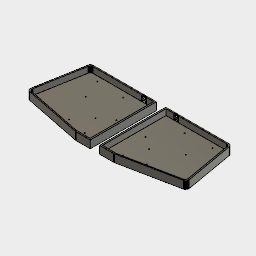
Split 62 bot (Autodesk Fusion 360 design; units mm, degrees)
Autodesk Fusion 360 part; units mm, degrees
note: some values were not read from the file. Chosen so that the rebuilt part matches the saved one: which pieces of a blend or face edit are solid. Set by a fixed rule: which sketch regions a step uses.
(part 1 of 2)
sketch "Sketch1" plane through (0, 0, 0) normal (0, 1, 0) x (1, 0, 0)
  line L0 (21.6572, -133.3169) -> (140.5792, -109.2975)
  line L1 (-8.8048, -133.4855) -> (-8.8048, 3.2554)
  line L2 (-8.8048, 3.2554) -> (-8.8048, -133.4855)
  line L3 (-8.8048, -133.4855) -> (20.1607, -133.4847)
  line L4 (20.1607, -133.4847) -> (20.9148, -133.4484)
  line L5 (20.9148, -133.4484) -> (20.9148, -133.4492)
  line L6 (20.9148, -133.4492) -> (21.658, -133.3177)
  line L7 (21.658, -133.3177) -> (140.5792, -109.2975)
  line L8 (140.5792, -109.2975) -> (141.2999, -109.074)
  line L9 (141.2999, -109.074) -> (141.9873, -108.7628)
  line L10 (141.9873, -108.7628) -> (141.9873, -108.7636)
  line L11 (141.9873, -108.7636) -> (142.6297, -108.368)
  line L12 (142.6297, -108.368) -> (142.6297, -108.3675)
  line L13 (142.6297, -108.3675) -> (143.2182, -107.8942)
  line L14 (143.2182, -107.8942) -> (143.2182, -107.8947)
  line L15 (143.2182, -107.8947) -> (143.7407, -107.3526)
  line L16 (143.7407, -107.3526) -> (143.742, -107.3518)
  line L17 (143.742, -107.3518) -> (144.1939, -106.7475)
  line L18 (144.1939, -106.7475) -> (144.567, -106.0918)
  line L19 (144.567, -106.0918) -> (144.8541, -105.3933)
  line L20 (144.8541, -105.3933) -> (145.0515, -104.6655)
  line L21 (145.0515, -104.6655) -> (145.0515, -104.6668)
  line L22 (145.0515, -104.6668) -> (145.157, -103.9196)
  line L23 (145.157, -103.9196) -> (145.1568, -103.9191)
  line L24 (145.1568, -103.9191) -> (145.1676, -103.1642)
  line L25 (145.1676, -103.1642) -> (145.1681, -103.165)
  line L26 (145.1681, -103.165) -> (145.0837, -102.4157)
  line L27 (145.0837, -102.4157) -> (127.3268, -1.7092)
  line L28 (127.3268, -1.7092) -> (127.1498, -0.9763)
  line L29 (127.1498, -0.9763) -> (126.8809, -0.2707)
  line L30 (126.8809, -0.2707) -> (126.5264, 0.3956)
  line L31 (126.5264, 0.3956) -> (126.0917, 1.0126)
  line L32 (126.0917, 1.0126) -> (125.584, 1.569)
  line L33 (125.584, 1.569) -> (125.5832, 1.569)
  line L34 (125.5832, 1.569) -> (125.008, 2.0577)
  line L35 (125.008, 2.0577) -> (124.3769, 2.4712)
  line L36 (124.3769, 2.4712) -> (123.698, 2.8022)
  line L37 (123.698, 2.8022) -> (122.9839, 3.0454)
  line L38 (122.9839, 3.0454) -> (122.9847, 3.0454)
  line L39 (122.9847, 3.0454) -> (122.2457, 3.1975)
  line L40 (122.2457, 3.1975) -> (121.4935, 3.2554)
  line L41 (-8.8048, 3.2554) -> (121.4935, 3.2554)
  line L42 (121.4935, 3.2554) -> (-8.8048, 3.2554)
  line L43 (20.9619, -101.3068) -> (36.3252, -98.5991)
  line L44 (36.3252, -98.5991) -> (34.1021, -85.9914)
  line L45 (34.1021, -85.9914) -> (18.7391, -88.7016)
  line L46 (18.7391, -88.7016) -> (20.9619, -101.3068)
  line L47 (17.6538, -82.5463) -> (33.0171, -79.8372)
  line L48 (33.0171, -79.8372) -> (30.7935, -67.233)
  line L49 (30.7935, -67.233) -> (15.4313, -69.9413)
  line L50 (15.4313, -69.9413) -> (17.6538, -82.5463)
  line L51 (14.3452, -63.7865) -> (29.709, -61.0775)
  line L52 (29.709, -61.0775) -> (27.4862, -48.4717)
  line L53 (27.4862, -48.4717) -> (12.1232, -51.1802)
  line L54 (12.1232, -51.1802) -> (14.3452, -63.7865)
  line L55 (11.0379, -45.0257) -> (26.4012, -42.3164)
  line L56 (26.4012, -42.3164) -> (24.1774, -29.7116)
  line L57 (24.1774, -29.7116) -> (8.8151, -32.4207)
  line L58 (8.8151, -32.4207) -> (11.0379, -45.0257)
  line L59 (24.3242, -119.9698) -> (39.6867, -117.2604)
  line L60 (39.6867, -117.2604) -> (37.4645, -104.6549)
  line L61 (37.4645, -104.6549) -> (22.1017, -107.3634)
  line L62 (22.1017, -107.3634) -> (24.3242, -119.9698)
  line L63 (38.8681, -92.991) -> (54.2311, -90.2819)
  line L64 (54.2311, -90.2819) -> (52.0084, -77.6764)
  line L65 (52.0084, -77.6764) -> (36.6453, -80.3857)
  line L66 (36.6453, -80.3857) -> (38.8681, -92.991)
  line L67 (35.4976, -74.2789) -> (50.8611, -71.5698)
  line L68 (50.8611, -71.5698) -> (48.6386, -58.965)
  line L69 (48.6386, -58.965) -> (33.2753, -61.6744)
  line L70 (33.2753, -61.6744) -> (35.4976, -74.2789)
  line L71 (32.2686, -55.5432) -> (47.6319, -52.8341)
  line L72 (47.6319, -52.8341) -> (45.4091, -40.2278)
  line L73 (45.4091, -40.2278) -> (30.0458, -42.9371)
  line L74 (30.0458, -42.9371) -> (32.2686, -55.5432)
  line L75 (28.8147, -36.8768) -> (44.1777, -34.1678)
  line L76 (44.1777, -34.1678) -> (41.9542, -21.563)
  line L77 (41.9542, -21.563) -> (26.5917, -24.2718)
  line L78 (26.5917, -24.2718) -> (28.8147, -36.8768)
  line L79 (42.1672, -111.7235) -> (57.5302, -109.0136)
  line L80 (57.5302, -109.0136) -> (55.3074, -96.4076)
  line L81 (55.3074, -96.4076) -> (39.9444, -99.1166)
  line L82 (39.9444, -99.1166) -> (42.1672, -111.7235)
  line L83 (56.5505, -83.8047) -> (71.9135, -81.0951)
  line L84 (71.9135, -81.0951) -> (69.6907, -68.489)
  line L85 (69.6907, -68.489) -> (54.3272, -71.1981)
  line L86 (54.3272, -71.1981) -> (56.5505, -83.8047)
  line L87 (53.2424, -65.1431) -> (68.6054, -62.4337)
  line L88 (68.6054, -62.4337) -> (66.3826, -49.8292)
  line L89 (66.3826, -49.8292) -> (51.0199, -52.5386)
  line L90 (51.0199, -52.5386) -> (53.2424, -65.1431)
  line L91 (49.9345, -46.383) -> (65.2973, -43.6742)
  line L92 (65.2973, -43.6742) -> (63.0748, -31.0679)
  line L93 (63.0748, -31.0679) -> (47.7118, -33.7772)
  line L94 (47.7118, -33.7772) -> (49.9345, -46.383)
  line L95 (46.6265, -27.6222) -> (61.9898, -24.9132)
  line L96 (61.9898, -24.9132) -> (59.7659, -12.3084)
  line L97 (59.7659, -12.3084) -> (44.4037, -15.0175)
  line L98 (44.4037, -15.0175) -> (46.6265, -27.6222)
  line L99 (59.7847, -102.5155) -> (75.1478, -99.8061)
  line L100 (75.1478, -99.8061) -> (72.925, -87.2001)
  line L101 (72.925, -87.2001) -> (57.5612, -89.9091)
  line L102 (57.5612, -89.9091) -> (59.7847, -102.5155)
  line L103 (76.1309, -85.4056) -> (91.494, -82.6966)
  line L104 (91.494, -82.6966) -> (89.2712, -70.091)
  line L105 (89.2712, -70.091) -> (73.9082, -72.8001)
  line L106 (73.9082, -72.8001) -> (76.1309, -85.4056)
  line L107 (72.8231, -66.6454) -> (88.1859, -63.9366)
  line L108 (88.1859, -63.9366) -> (85.9634, -51.3313)
  line L109 (85.9634, -51.3313) -> (70.5996, -54.0406)
  line L110 (70.5996, -54.0406) -> (72.8231, -66.6454)
  line L111 (69.515, -47.8859) -> (84.8781, -45.1765)
  line L112 (84.8781, -45.1765) -> (82.6553, -32.5705)
  line L113 (82.6553, -32.5705) -> (67.2917, -35.2795)
  line L114 (67.2917, -35.2795) -> (69.515, -47.8859)
  line L115 (66.207, -29.2428) -> (81.57, -26.534)
  line L116 (81.57, -26.534) -> (79.3467, -13.9287)
  line L117 (79.3467, -13.9287) -> (63.9837, -16.6373)
  line L118 (63.9837, -16.6373) -> (66.207, -29.2428)
  line L119 (79.3644, -104.2064) -> (94.7277, -101.4965)
  line L120 (94.7277, -101.4965) -> (92.5049, -88.8899)
  line L121 (92.5049, -88.8899) -> (77.1417, -91.6001)
  line L122 (77.1417, -91.6001) -> (79.3644, -104.2064)
  line L123 (95.3622, -85.0606) -> (110.7252, -82.3516)
  line L124 (110.7252, -82.3516) -> (108.5025, -69.745)
  line L125 (108.5025, -69.745) -> (93.1394, -72.4543)
  line L126 (93.1394, -72.4543) -> (95.3622, -85.0606)
  line L127 (92.0541, -66.2993) -> (107.4174, -63.5908)
  line L128 (107.4174, -63.5908) -> (105.1944, -50.9857)
  line L129 (105.1944, -50.9857) -> (89.8313, -53.6948)
  line L130 (89.8313, -53.6948) -> (92.0541, -66.2993)
  line L131 (88.746, -47.5401) -> (104.1093, -44.8302)
  line L132 (104.1093, -44.8302) -> (101.8865, -32.2247)
  line L133 (101.8865, -32.2247) -> (86.5235, -34.9337)
  line L134 (86.5235, -34.9337) -> (88.746, -47.5401)
  line L135 (85.4385, -28.8973) -> (100.8012, -26.1885)
  line L136 (100.8012, -26.1885) -> (98.5787, -13.5834)
  line L137 (98.5787, -13.5834) -> (83.2154, -16.2925)
  line L138 (83.2154, -16.2925) -> (85.4385, -28.8973)
  line L139 (98.5965, -103.8611) -> (113.9587, -101.1513)
  line L140 (113.9587, -101.1513) -> (111.7367, -88.5449)
  line L141 (111.7367, -88.5449) -> (96.3737, -91.2543)
  line L142 (96.3737, -91.2543) -> (98.5965, -103.8611)
  line L143 (114.0738, -81.6816) -> (129.4368, -78.9723)
  line L144 (129.4368, -78.9723) -> (127.214, -66.3662)
  line L145 (127.214, -66.3662) -> (111.8513, -69.0753)
  line L146 (111.8513, -69.0753) -> (114.0738, -81.6816)
  line L147 (110.766, -62.9211) -> (126.129, -60.2123)
  line L148 (126.129, -60.2123) -> (123.9062, -47.607)
  line L149 (123.9062, -47.607) -> (108.5432, -50.3163)
  line L150 (108.5432, -50.3163) -> (110.766, -62.9211)
  line L151 (107.4579, -44.3008) -> (122.8212, -41.5917)
  line L152 (122.8212, -41.5917) -> (120.5981, -28.9859)
  line L153 (120.5981, -28.9859) -> (105.2351, -31.695)
  line L154 (105.2351, -31.695) -> (107.4579, -44.3008)
  line L155 (104.2464, -25.5889) -> (119.6094, -22.8804)
  line L156 (119.6094, -22.8804) -> (117.3861, -10.2754)
  line L157 (117.3861, -10.2754) -> (102.0236, -12.9842)
  line L158 (102.0236, -12.9842) -> (104.2464, -25.5889)
  line L159 (117.3075, -100.4816) -> (132.6706, -97.7731)
  line L160 (132.6706, -97.7731) -> (130.4478, -85.1659)
  line L161 (130.4478, -85.1659) -> (115.0845, -87.875)
  line L162 (115.0845, -87.875) -> (117.3075, -100.4816)
  line L163 (3.9632, -113.914) -> (19.326, -111.2038)
  line L164 (19.326, -111.2038) -> (17.1035, -98.5986)
  line L165 (17.1035, -98.5986) -> (1.7404, -101.3063)
  line L166 (1.7404, -101.3063) -> (3.9632, -113.914)
  line L167 (19.6816, -136.2128) -> (143.6531, -111.1734)
  line L168 (-12.0737, -136.3885) -> (-12.0737, 6.1587)
  line L169 (-12.0737, 6.1587) -> (-12.0737, -136.3885)
  line L170 (-12.0737, -136.3885) -> (18.1216, -136.3877)
  line L171 (18.1216, -136.3877) -> (18.9079, -136.3493)
  line L172 (18.9079, -136.3493) -> (18.9079, -136.3501)
  line L173 (18.9079, -136.3501) -> (19.6824, -136.2139)
  line L174 (19.6824, -136.2139) -> (143.6531, -111.1734)
  line L175 (143.6531, -111.1734) -> (144.4046, -110.9403)
  line L176 (144.4046, -110.9403) -> (145.121, -110.6159)
  line L177 (145.121, -110.6159) -> (145.121, -110.6167)
  line L178 (145.121, -110.6167) -> (145.7907, -110.2045)
  line L179 (145.7907, -110.2045) -> (145.7907, -110.204)
  line L180 (145.7907, -110.204) -> (146.4043, -109.7103)
  line L181 (146.4043, -109.7103) -> (146.4043, -109.7113)
  line L182 (146.4043, -109.7113) -> (146.9488, -109.1457)
  line L183 (146.9488, -109.1457) -> (146.9501, -109.1449)
  line L184 (146.9501, -109.1449) -> (147.4213, -108.5146)
  line L185 (147.4213, -108.5146) -> (147.8108, -107.8315)
  line L186 (147.8108, -107.8315) -> (148.1098, -107.1036)
  line L187 (148.1098, -107.1036) -> (148.3154, -106.3448)
  line L188 (148.3154, -106.3448) -> (148.3154, -106.3461)
  line L189 (148.3154, -106.3461) -> (148.4257, -105.5672)
  line L190 (148.4257, -105.5672) -> (148.4249, -105.5666)
  line L191 (148.4249, -105.5666) -> (148.4363, -104.7795)
  line L192 (148.4363, -104.7795) -> (148.4371, -104.7803)
  line L193 (148.4371, -104.7803) -> (148.3492, -103.9992)
  line L194 (148.3492, -103.9992) -> (129.8382, 0.9829)
  line L195 (129.8382, 0.9829) -> (129.6532, 1.7473)
  line L196 (129.6532, 1.7473) -> (129.3736, 2.4831)
  line L197 (129.3736, 2.4831) -> (129.004, 3.1771)
  line L198 (129.004, 3.1771) -> (128.5505, 3.8201)
  line L199 (128.5505, 3.8201) -> (128.0213, 4.4006)
  line L200 (128.0213, 4.4006) -> (128.0208, 4.4006)
  line L201 (128.0208, 4.4006) -> (127.4204, 4.9101)
  line L202 (127.4204, 4.9101) -> (126.7632, 5.3411)
  line L203 (126.7632, 5.3411) -> (126.0554, 5.6864)
  line L204 (126.0554, 5.6864) -> (125.3112, 5.9396)
  line L205 (125.3112, 5.9396) -> (125.312, 5.9396)
  line L206 (125.312, 5.9396) -> (124.5415, 6.0984)
  line L207 (124.5415, 6.0984) -> (123.7575, 6.1587)
  line L208 (-12.0737, 6.1587) -> (123.7575, 6.1587)
  line L209 (123.7575, 6.1587) -> (-12.0737, 6.1587)
extrude "Extrude1" add sketch "Sketch1" along normal blind 16.7 contours L167 L168 L169 L170 L171 L173 L174 L175 L176 L178 L180 L182 L184 L185 L186 L187 L189 L191 L193 L194 L195 L196 L197 L198 L199 L201 L202 L203 L204 L206 L207 L208 L209 makes body 1
sketch "Sketch2" plane through (0, 0, 0) normal (0, 1, 0) x (1, 0, 0)
  line L0 (21.6572, -133.3169) -> (140.5792, -109.2975)
  line L1 (-8.8048, -133.4855) -> (-8.8048, 3.2554)
  line L2 (-8.8048, 3.2554) -> (-8.8048, -133.4855)
  line L3 (-8.8048, -133.4855) -> (20.1607, -133.4847)
  line L4 (20.1607, -133.4847) -> (20.9148, -133.4484)
  line L5 (20.9148, -133.4484) -> (20.9148, -133.4492)
  line L6 (20.9148, -133.4492) -> (21.658, -133.3177)
  line L7 (21.658, -133.3177) -> (140.5792, -109.2975)
  line L8 (140.5792, -109.2975) -> (141.2999, -109.074)
  line L9 (141.2999, -109.074) -> (141.9873, -108.7628)
  line L10 (141.9873, -108.7628) -> (141.9873, -108.7636)
  line L11 (141.9873, -108.7636) -> (142.6297, -108.368)
  line L12 (142.6297, -108.368) -> (142.6297, -108.3675)
  line L13 (142.6297, -108.3675) -> (143.2182, -107.8942)
  line L14 (143.2182, -107.8942) -> (143.2182, -107.8947)
  line L15 (143.2182, -107.8947) -> (143.7407, -107.3526)
  line L16 (143.7407, -107.3526) -> (143.742, -107.3518)
  line L17 (143.742, -107.3518) -> (144.1939, -106.7475)
  line L18 (144.1939, -106.7475) -> (144.567, -106.0918)
  line L19 (144.567, -106.0918) -> (144.8541, -105.3933)
  line L20 (144.8541, -105.3933) -> (145.0515, -104.6655)
  line L21 (145.0515, -104.6655) -> (145.0515, -104.6668)
  line L22 (145.0515, -104.6668) -> (145.157, -103.9196)
  line L23 (145.157, -103.9196) -> (145.1568, -103.9191)
  line L24 (145.1568, -103.9191) -> (145.1676, -103.1642)
  line L25 (145.1676, -103.1642) -> (145.1681, -103.165)
  line L26 (145.1681, -103.165) -> (145.0837, -102.4157)
  line L27 (145.0837, -102.4157) -> (127.3268, -1.7092)
  line L28 (127.3268, -1.7092) -> (127.1498, -0.9763)
  line L29 (127.1498, -0.9763) -> (126.8809, -0.2707)
  line L30 (126.8809, -0.2707) -> (126.5264, 0.3956)
  line L31 (126.5264, 0.3956) -> (126.0917, 1.0126)
  line L32 (126.0917, 1.0126) -> (125.584, 1.569)
  line L33 (125.584, 1.569) -> (125.5832, 1.569)
  line L34 (125.5832, 1.569) -> (125.008, 2.0577)
  line L35 (125.008, 2.0577) -> (124.3769, 2.4712)
  line L36 (124.3769, 2.4712) -> (123.698, 2.8022)
  line L37 (123.698, 2.8022) -> (122.9839, 3.0454)
  line L38 (122.9839, 3.0454) -> (122.9847, 3.0454)
  line L39 (122.9847, 3.0454) -> (122.2457, 3.1975)
  line L40 (122.2457, 3.1975) -> (121.4935, 3.2554)
  line L41 (-8.8048, 3.2554) -> (121.4935, 3.2554)
  line L42 (121.4935, 3.2554) -> (-8.8048, 3.2554)
  line L43 (20.9619, -101.3068) -> (36.3252, -98.5991)
  line L44 (36.3252, -98.5991) -> (34.1021, -85.9914)
  line L45 (34.1021, -85.9914) -> (18.7391, -88.7016)
  line L46 (18.7391, -88.7016) -> (20.9619, -101.3068)
  line L47 (17.6538, -82.5463) -> (33.0171, -79.8372)
  line L48 (33.0171, -79.8372) -> (30.7935, -67.233)
  line L49 (30.7935, -67.233) -> (15.4313, -69.9413)
  line L50 (15.4313, -69.9413) -> (17.6538, -82.5463)
  line L51 (14.3452, -63.7865) -> (29.709, -61.0775)
  line L52 (29.709, -61.0775) -> (27.4862, -48.4717)
  line L53 (27.4862, -48.4717) -> (12.1232, -51.1802)
  line L54 (12.1232, -51.1802) -> (14.3452, -63.7865)
  line L55 (11.0379, -45.0257) -> (26.4012, -42.3164)
  line L56 (26.4012, -42.3164) -> (24.1774, -29.7116)
  line L57 (24.1774, -29.7116) -> (8.8151, -32.4207)
  line L58 (8.8151, -32.4207) -> (11.0379, -45.0257)
  line L59 (24.3242, -119.9698) -> (39.6867, -117.2604)
  line L60 (39.6867, -117.2604) -> (37.4645, -104.6549)
  line L61 (37.4645, -104.6549) -> (22.1017, -107.3634)
  line L62 (22.1017, -107.3634) -> (24.3242, -119.9698)
  line L63 (38.8681, -92.991) -> (54.2311, -90.2819)
  line L64 (54.2311, -90.2819) -> (52.0084, -77.6764)
  line L65 (52.0084, -77.6764) -> (36.6453, -80.3857)
  line L66 (36.6453, -80.3857) -> (38.8681, -92.991)
  line L67 (35.4976, -74.2789) -> (50.8611, -71.5698)
  line L68 (50.8611, -71.5698) -> (48.6386, -58.965)
  line L69 (48.6386, -58.965) -> (33.2753, -61.6744)
  line L70 (33.2753, -61.6744) -> (35.4976, -74.2789)
  line L71 (32.2686, -55.5432) -> (47.6319, -52.8341)
  line L72 (47.6319, -52.8341) -> (45.4091, -40.2278)
  line L73 (45.4091, -40.2278) -> (30.0458, -42.9371)
  line L74 (30.0458, -42.9371) -> (32.2686, -55.5432)
  line L75 (28.8147, -36.8768) -> (44.1777, -34.1678)
  line L76 (44.1777, -34.1678) -> (41.9542, -21.563)
  line L77 (41.9542, -21.563) -> (26.5917, -24.2718)
  line L78 (26.5917, -24.2718) -> (28.8147, -36.8768)
  line L79 (42.1672, -111.7235) -> (57.5302, -109.0136)
  line L80 (57.5302, -109.0136) -> (55.3074, -96.4076)
  line L81 (55.3074, -96.4076) -> (39.9444, -99.1166)
  line L82 (39.9444, -99.1166) -> (42.1672, -111.7235)
  line L83 (56.5505, -83.8047) -> (71.9135, -81.0951)
  line L84 (71.9135, -81.0951) -> (69.6907, -68.489)
  line L85 (69.6907, -68.489) -> (54.3272, -71.1981)
  line L86 (54.3272, -71.1981) -> (56.5505, -83.8047)
  line L87 (53.2424, -65.1431) -> (68.6054, -62.4337)
  line L88 (68.6054, -62.4337) -> (66.3826, -49.8292)
  line L89 (66.3826, -49.8292) -> (51.0199, -52.5386)
  line L90 (51.0199, -52.5386) -> (53.2424, -65.1431)
  line L91 (49.9345, -46.383) -> (65.2973, -43.6742)
  line L92 (65.2973, -43.6742) -> (63.0748, -31.0679)
  line L93 (63.0748, -31.0679) -> (47.7118, -33.7772)
  line L94 (47.7118, -33.7772) -> (49.9345, -46.383)
  line L95 (46.6265, -27.6222) -> (61.9898, -24.9132)
  line L96 (61.9898, -24.9132) -> (59.7659, -12.3084)
  line L97 (59.7659, -12.3084) -> (44.4037, -15.0175)
  line L98 (44.4037, -15.0175) -> (46.6265, -27.6222)
  line L99 (59.7847, -102.5155) -> (75.1478, -99.8061)
  line L100 (75.1478, -99.8061) -> (72.925, -87.2001)
  line L101 (72.925, -87.2001) -> (57.5612, -89.9091)
  line L102 (57.5612, -89.9091) -> (59.7847, -102.5155)
  line L103 (76.1309, -85.4056) -> (91.494, -82.6966)
  line L104 (91.494, -82.6966) -> (89.2712, -70.091)
  line L105 (89.2712, -70.091) -> (73.9082, -72.8001)
  line L106 (73.9082, -72.8001) -> (76.1309, -85.4056)
  line L107 (72.8231, -66.6454) -> (88.1859, -63.9366)
  line L108 (88.1859, -63.9366) -> (85.9634, -51.3313)
  line L109 (85.9634, -51.3313) -> (70.5996, -54.0406)
  line L110 (70.5996, -54.0406) -> (72.8231, -66.6454)
  line L111 (69.515, -47.8859) -> (84.8781, -45.1765)
  line L112 (84.8781, -45.1765) -> (82.6553, -32.5705)
  line L113 (82.6553, -32.5705) -> (67.2917, -35.2795)
  line L114 (67.2917, -35.2795) -> (69.515, -47.8859)
  line L115 (66.207, -29.2428) -> (81.57, -26.534)
  line L116 (81.57, -26.534) -> (79.3467, -13.9287)
  line L117 (79.3467, -13.9287) -> (63.9837, -16.6373)
  line L118 (63.9837, -16.6373) -> (66.207, -29.2428)
  line L119 (79.3644, -104.2064) -> (94.7277, -101.4965)
  line L120 (94.7277, -101.4965) -> (92.5049, -88.8899)
  line L121 (92.5049, -88.8899) -> (77.1417, -91.6001)
  line L122 (77.1417, -91.6001) -> (79.3644, -104.2064)
  line L123 (95.3622, -85.0606) -> (110.7252, -82.3516)
  line L124 (110.7252, -82.3516) -> (108.5025, -69.745)
  line L125 (108.5025, -69.745) -> (93.1394, -72.4543)
  line L126 (93.1394, -72.4543) -> (95.3622, -85.0606)
  line L127 (92.0541, -66.2993) -> (107.4174, -63.5908)
  line L128 (107.4174, -63.5908) -> (105.1944, -50.9857)
  line L129 (105.1944, -50.9857) -> (89.8313, -53.6948)
  line L130 (89.8313, -53.6948) -> (92.0541, -66.2993)
  line L131 (88.746, -47.5401) -> (104.1093, -44.8302)
  line L132 (104.1093, -44.8302) -> (101.8865, -32.2247)
  line L133 (101.8865, -32.2247) -> (86.5235, -34.9337)
  line L134 (86.5235, -34.9337) -> (88.746, -47.5401)
  line L135 (85.4385, -28.8973) -> (100.8012, -26.1885)
  line L136 (100.8012, -26.1885) -> (98.5787, -13.5834)
  line L137 (98.5787, -13.5834) -> (83.2154, -16.2925)
  line L138 (83.2154, -16.2925) -> (85.4385, -28.8973)
  line L139 (98.5965, -103.8611) -> (113.9587, -101.1513)
  line L140 (113.9587, -101.1513) -> (111.7367, -88.5449)
  line L141 (111.7367, -88.5449) -> (96.3737, -91.2543)
  line L142 (96.3737, -91.2543) -> (98.5965, -103.8611)
  line L143 (114.0738, -81.6816) -> (129.4368, -78.9723)
  line L144 (129.4368, -78.9723) -> (127.214, -66.3662)
  line L145 (127.214, -66.3662) -> (111.8513, -69.0753)
  line L146 (111.8513, -69.0753) -> (114.0738, -81.6816)
  line L147 (110.766, -62.9211) -> (126.129, -60.2123)
  line L148 (126.129, -60.2123) -> (123.9062, -47.607)
  line L149 (123.9062, -47.607) -> (108.5432, -50.3163)
  line L150 (108.5432, -50.3163) -> (110.766, -62.9211)
  line L151 (107.4579, -44.3008) -> (122.8212, -41.5917)
  line L152 (122.8212, -41.5917) -> (120.5981, -28.9859)
  line L153 (120.5981, -28.9859) -> (105.2351, -31.695)
  line L154 (105.2351, -31.695) -> (107.4579, -44.3008)
  line L155 (104.2464, -25.5889) -> (119.6094, -22.8804)
  line L156 (119.6094, -22.8804) -> (117.3861, -10.2754)
  line L157 (117.3861, -10.2754) -> (102.0236, -12.9842)
  line L158 (102.0236, -12.9842) -> (104.2464, -25.5889)
  line L159 (117.3075, -100.4816) -> (132.6706, -97.7731)
  line L160 (132.6706, -97.7731) -> (130.4478, -85.1659)
  line L161 (130.4478, -85.1659) -> (115.0845, -87.875)
  line L162 (115.0845, -87.875) -> (117.3075, -100.4816)
  line L163 (3.9632, -113.914) -> (19.326, -111.2038)
  line L164 (19.326, -111.2038) -> (17.1035, -98.5986)
  line L165 (17.1035, -98.5986) -> (1.7404, -101.3063)
  line L166 (1.7404, -101.3063) -> (3.9632, -113.914)
  line L167 (19.6816, -136.2128) -> (143.6531, -111.1734)
  line L168 (-12.0737, -136.3885) -> (-12.0737, 6.1587)
  line L169 (-12.0737, 6.1587) -> (-12.0737, -136.3885)
  line L170 (-12.0737, -136.3885) -> (18.1216, -136.3877)
  line L171 (18.1216, -136.3877) -> (18.9079, -136.3493)
  line L172 (18.9079, -136.3493) -> (18.9079, -136.3501)
  line L173 (18.9079, -136.3501) -> (19.6824, -136.2139)
  line L174 (19.6824, -136.2139) -> (143.6531, -111.1734)
  line L175 (143.6531, -111.1734) -> (144.4046, -110.9403)
  line L176 (144.4046, -110.9403) -> (145.121, -110.6159)
  line L177 (145.121, -110.6159) -> (145.121, -110.6167)
  line L178 (145.121, -110.6167) -> (145.7907, -110.2045)
  line L179 (145.7907, -110.2045) -> (145.7907, -110.204)
  line L180 (145.7907, -110.204) -> (146.4043, -109.7103)
  line L181 (146.4043, -109.7103) -> (146.4043, -109.7113)
  line L182 (146.4043, -109.7113) -> (146.9488, -109.1457)
  line L183 (146.9488, -109.1457) -> (146.9501, -109.1449)
  line L184 (146.9501, -109.1449) -> (147.4213, -108.5146)
  line L185 (147.4213, -108.5146) -> (147.8108, -107.8315)
  line L186 (147.8108, -107.8315) -> (148.1098, -107.1036)
  line L187 (148.1098, -107.1036) -> (148.3154, -106.3448)
  line L188 (148.3154, -106.3448) -> (148.3154, -106.3461)
  line L189 (148.3154, -106.3461) -> (148.4257, -105.5672)
  line L190 (148.4257, -105.5672) -> (148.4249, -105.5666)
  line L191 (148.4249, -105.5666) -> (148.4363, -104.7795)
  line L192 (148.4363, -104.7795) -> (148.4371, -104.7803)
  line L193 (148.4371, -104.7803) -> (148.3492, -103.9992)
  line L194 (148.3492, -103.9992) -> (129.8382, 0.9829)
  line L195 (129.8382, 0.9829) -> (129.6532, 1.7473)
  line L196 (129.6532, 1.7473) -> (129.3736, 2.4831)
  line L197 (129.3736, 2.4831) -> (129.004, 3.1771)
  line L198 (129.004, 3.1771) -> (128.5505, 3.8201)
  line L199 (128.5505, 3.8201) -> (128.0213, 4.4006)
  line L200 (128.0213, 4.4006) -> (128.0208, 4.4006)
  line L201 (128.0208, 4.4006) -> (127.4204, 4.9101)
  line L202 (127.4204, 4.9101) -> (126.7632, 5.3411)
  line L203 (126.7632, 5.3411) -> (126.0554, 5.6864)
  line L204 (126.0554, 5.6864) -> (125.3112, 5.9396)
  line L205 (125.3112, 5.9396) -> (125.312, 5.9396)
  line L206 (125.312, 5.9396) -> (124.5415, 6.0984)
  line L207 (124.5415, 6.0984) -> (123.7575, 6.1587)
  line L208 (-12.0737, 6.1587) -> (123.7575, 6.1587)
  line L209 (123.7575, 6.1587) -> (-12.0737, 6.1587)
extrude "Extrude2" add sketch "Sketch2" along normal blind 4 contours L0 L1 L2 L3 L4 L6 L7 L8 L9 L11 L13 L15 L17 L18 L19 L20 L22 L24 L26 L27 L28 L29 L30 L31 L32 L34 L35 L36 L37 L39 L40 L41 L42 | L43 L44 L45 L46 | L47 L48 L49 L50 | L51 L52 L53 L54 | L55 L56 L57 L58 | L59 L60 L61 L62 | L63 L64 L65 L66 | L67 L68 L69 L70 | L71 L72 L73 L74 | L75 L76 L77 L78 | L79 L80 L81 L82 | L83 L84 L85 L86 | L87 L88 L89 L90 | L91 L92 L93 L94 | L95 L96 L97 L98 | L99 L100 L101 L102 | L103 L104 L105 L106 | L107 L108 L109 L110 | L111 L112 L113 L114 | L115 L116 L117 L118 | L119 L120 L121 L122 | L123 L124 L125 L126 | L127 L128 L129 L130 | L131 L132 L133 L134 | L135 L136 L137 L138 | L139 L140 L141 L142 | L143 L144 L145 L146 | L147 L148 L149 L150 | L151 L152 L153 L154 | L155 L156 L157 L158 | L159 L160 L161 L162 | L163 L164 L165 L166 bodies 1
sketch "Sketch4" plane through (0, 4, 0) normal (0, 1, 0) x (-1, 0, 0)
  line L0 (-121.4935, -3.2554) -> (8.8048, -3.2554)
  line L1 (8.8048, -3.2554) -> (8.8048, 133.4855)
  line L2 (8.8048, 133.4855) -> (-20.1607, 133.4847)
  line L3 (-20.1607, 133.4847) -> (-20.9148, 133.4484)
  line L4 (-20.9148, 133.4484) -> (-20.9148, 133.4492)
  line L5 (-20.9148, 133.4492) -> (-21.658, 133.3177)
  line L6 (-21.658, 133.3177) -> (-140.5792, 109.2975)
  line L7 (-140.5792, 109.2975) -> (-141.2999, 109.074)
  line L8 (-141.2999, 109.074) -> (-141.9873, 108.7628)
  line L9 (-141.9873, 108.7628) -> (-141.9873, 108.7636)
  line L10 (-141.9873, 108.7636) -> (-142.6297, 108.368)
  line L11 (-142.6297, 108.368) -> (-142.6297, 108.3675)
  line L12 (-142.6297, 108.3675) -> (-143.2182, 107.8942)
  line L13 (-143.2182, 107.8942) -> (-143.2182, 107.8947)
  line L14 (-143.2182, 107.8947) -> (-143.7407, 107.3526)
  line L15 (-143.7407, 107.3526) -> (-143.742, 107.3518)
  line L16 (-143.742, 107.3518) -> (-144.1939, 106.7475)
  line L17 (-144.1939, 106.7475) -> (-144.567, 106.0918)
  line L18 (-144.567, 106.0918) -> (-144.8541, 105.3933)
  line L19 (-144.8541, 105.3933) -> (-145.0515, 104.6655)
  line L20 (-145.0515, 104.6655) -> (-145.0515, 104.6668)
  line L21 (-145.0515, 104.6668) -> (-145.157, 103.9196)
  line L22 (-145.157, 103.9196) -> (-145.1568, 103.9191)
  line L23 (-145.1568, 103.9191) -> (-145.1676, 103.1642)
  line L24 (-145.1676, 103.1642) -> (-145.1681, 103.165)
  line L25 (-145.1681, 103.165) -> (-145.0837, 102.4157)
  line L26 (-145.0837, 102.4157) -> (-127.3268, 1.7092)
  line L27 (-127.3268, 1.7092) -> (-127.1498, 0.9763)
  line L28 (-127.1498, 0.9763) -> (-126.8809, 0.2707)
  line L29 (-126.8809, 0.2707) -> (-126.5264, -0.3956)
  line L30 (-126.5264, -0.3956) -> (-126.0917, -1.0126)
  line L31 (-126.0917, -1.0126) -> (-125.584, -1.569)
  line L32 (-125.584, -1.569) -> (-125.5832, -1.569)
  line L33 (-125.5832, -1.569) -> (-125.008, -2.0577)
  line L34 (-125.008, -2.0577) -> (-124.3769, -2.4712)
  line L35 (-124.3769, -2.4712) -> (-123.698, -2.8022)
  line L36 (-123.698, -2.8022) -> (-122.9839, -3.0454)
  line L37 (-122.9839, -3.0454) -> (-122.9847, -3.0454)
  line L38 (-122.9847, -3.0454) -> (-122.2457, -3.1975)
  line L39 (-122.2457, -3.1975) -> (-121.4935, -3.2554)
  line L40 (12.0737, -6.1587) -> (12.0737, -0.9787)
  line L41 (12.0737, -0.9787) -> (-1.0193, -0.9787)
  circle A0 centre (-1.0193, 0.1713) radius 1.15
  line L42 (-2.1693, 0.1713) -> (-15.2793, 0.1713)
  circle A1 centre (-16.4293, 0.1713) radius 1.15
  point P0 (12.0737, -6.1587)
  dimension "d7" = 5.18
  dimension "d8" = 13.093
  dimension "d9" = 2.3
  dimension "d10" = 13.11
  dimension "d11" = 2.3
  measures "d7" distance of P0 L40.end
  measures "d8" distance of L40.end L41.end
  measures "d9" diameter of A0
  measures "d10" distance of L42.start L42.end
  measures "d11" diameter of A1
extrude "Extrude4" cut sketch "Sketch4" against normal blind 5 contours A0 | A1 bodies 1
sketch "Sketch5" plane through (0, 4, 0) normal (0, 1, 0) x (-1, 0, 0)
  circle A0 centre (-1.0193, 0.1713) radius 1.15
  circle A1 centre (-16.4293, 0.1713) radius 1.15
  line L0 (-121.4935, -3.2554) -> (8.8048, -3.2554)
  line L1 (8.8048, -3.2554) -> (8.8048, 133.4855)
  line L2 (8.8048, 133.4855) -> (-20.1607, 133.4847)
  line L3 (-20.1607, 133.4847) -> (-20.9148, 133.4484)
  line L4 (-20.9148, 133.4484) -> (-20.9148, 133.4492)
  line L5 (-20.9148, 133.4492) -> (-21.658, 133.3177)
  line L6 (-21.658, 133.3177) -> (-140.5792, 109.2975)
  line L7 (-140.5792, 109.2975) -> (-141.2999, 109.074)
  line L8 (-141.2999, 109.074) -> (-141.9873, 108.7628)
  line L9 (-141.9873, 108.7628) -> (-141.9873, 108.7636)
  line L10 (-141.9873, 108.7636) -> (-142.6297, 108.368)
  line L11 (-142.6297, 108.368) -> (-142.6297, 108.3675)
  line L12 (-142.6297, 108.3675) -> (-143.2182, 107.8942)
  line L13 (-143.2182, 107.8942) -> (-143.2182, 107.8947)
  line L14 (-143.2182, 107.8947) -> (-143.7407, 107.3526)
  line L15 (-143.7407, 107.3526) -> (-143.742, 107.3518)
  line L16 (-143.742, 107.3518) -> (-144.1939, 106.7475)
  line L17 (-144.1939, 106.7475) -> (-144.567, 106.0918)
  line L18 (-144.567, 106.0918) -> (-144.8541, 105.3933)
  line L19 (-144.8541, 105.3933) -> (-145.0515, 104.6655)
  line L20 (-145.0515, 104.6655) -> (-145.0515, 104.6668)
  line L21 (-145.0515, 104.6668) -> (-145.157, 103.9196)
  line L22 (-145.157, 103.9196) -> (-145.1568, 103.9191)
  line L23 (-145.1568, 103.9191) -> (-145.1676, 103.1642)
  line L24 (-145.1676, 103.1642) -> (-145.1681, 103.165)
  line L25 (-145.1681, 103.165) -> (-145.0837, 102.4157)
  line L26 (-145.0837, 102.4157) -> (-127.3268, 1.7092)
  line L27 (-127.3268, 1.7092) -> (-127.1498, 0.9763)
  line L28 (-127.1498, 0.9763) -> (-126.8809, 0.2707)
  line L29 (-126.8809, 0.2707) -> (-126.5264, -0.3956)
  line L30 (-126.5264, -0.3956) -> (-126.0917, -1.0126)
  line L31 (-126.0917, -1.0126) -> (-125.584, -1.569)
  line L32 (-125.584, -1.569) -> (-125.5832, -1.569)
  line L33 (-125.5832, -1.569) -> (-125.008, -2.0577)
  line L34 (-125.008, -2.0577) -> (-124.3769, -2.4712)
  line L35 (-124.3769, -2.4712) -> (-123.698, -2.8022)
  line L36 (-123.698, -2.8022) -> (-122.9839, -3.0454)
  line L37 (-122.9839, -3.0454) -> (-122.9847, -3.0454)
  line L38 (-122.9847, -3.0454) -> (-122.2457, -3.1975)
  line L39 (-122.2457, -3.1975) -> (-121.4935, -3.2554)
  line L40 (-20.9616, 101.3071) -> (-36.3252, 98.5991)
  line L41 (-36.3252, 98.5991) -> (-34.1019, 85.9917)
  line L42 (-34.1019, 85.9917) -> (-18.7391, 88.701)
  line L43 (-18.7391, 88.701) -> (-20.9616, 101.3071)
  line L44 (-17.6538, 82.5463) -> (-33.0171, 79.837)
  line L45 (-33.0171, 79.837) -> (-30.7933, 67.233)
  line L46 (-30.7933, 67.233) -> (-15.4313, 69.9415)
  line L47 (-15.4313, 69.9415) -> (-17.6538, 82.5463)
  line L48 (-14.3449, 63.7865) -> (-29.709, 61.0775)
  line L49 (-29.709, 61.0775) -> (-27.486, 48.4714)
  line L50 (-27.486, 48.4714) -> (-12.1235, 51.1802)
  line L51 (-12.1235, 51.1802) -> (-14.3449, 63.7865)
  line L52 (-11.0376, 45.0257) -> (-26.4012, 42.3164)
  line L53 (-26.4012, 42.3164) -> (-24.1774, 29.7116)
  line L54 (-24.1774, 29.7116) -> (-8.8154, 32.4207)
  line L55 (-8.8154, 32.4207) -> (-11.0376, 45.0257)
  line L56 (-24.3245, 119.9695) -> (-39.6867, 117.2602)
  line L57 (-39.6867, 117.2602) -> (-37.4647, 104.6551)
  line L58 (-37.4647, 104.6551) -> (-22.1017, 107.3634)
  line L59 (-22.1017, 107.3634) -> (-24.3245, 119.9695)
  line L60 (-38.8681, 92.9913) -> (-54.2311, 90.2819)
  line L61 (-54.2311, 90.2819) -> (-52.0084, 77.6758)
  line L62 (-52.0084, 77.6758) -> (-36.6451, 80.3857)
  line L63 (-36.6451, 80.3857) -> (-38.8681, 92.9913)
  line L64 (-35.4973, 74.2786) -> (-50.8611, 71.5698)
  line L65 (-50.8611, 71.5698) -> (-48.6384, 58.9648)
  line L66 (-48.6384, 58.9648) -> (-33.2756, 61.6744)
  line L67 (-33.2756, 61.6744) -> (-35.4973, 74.2786)
  line L68 (-32.2686, 55.5432) -> (-47.6319, 52.8341)
  line L69 (-47.6319, 52.8341) -> (-45.4091, 40.2278)
  line L70 (-45.4091, 40.2278) -> (-30.0458, 42.9368)
  line L71 (-30.0458, 42.9368) -> (-32.2686, 55.5432)
  line L72 (-28.8147, 36.8768) -> (-44.1777, 34.1675)
  line L73 (-44.1777, 34.1675) -> (-41.9542, 21.5625)
  line L74 (-41.9542, 21.5625) -> (-26.5917, 24.2718)
  line L75 (-26.5917, 24.2718) -> (-28.8147, 36.8768)
  line L76 (-42.1674, 111.7235) -> (-57.5299, 109.0136)
  line L77 (-57.5299, 109.0136) -> (-55.3077, 96.4076)
  line L78 (-55.3077, 96.4076) -> (-39.9444, 99.1164)
  line L79 (-39.9444, 99.1164) -> (-42.1674, 111.7235)
  line L80 (-56.5505, 83.8047) -> (-71.9135, 81.0953)
  line L81 (-71.9135, 81.0953) -> (-69.6907, 68.4887)
  line L82 (-69.6907, 68.4887) -> (-54.3269, 71.1983)
  line L83 (-54.3269, 71.1983) -> (-56.5505, 83.8047)
  line L84 (-53.2424, 65.1431) -> (-68.6054, 62.4335)
  line L85 (-68.6054, 62.4335) -> (-66.3826, 49.829)
  line L86 (-66.3826, 49.829) -> (-51.0196, 52.5386)
  line L87 (-51.0196, 52.5386) -> (-53.2424, 65.1431)
  line L88 (-49.9345, 46.3828) -> (-65.2973, 43.6742)
  line L89 (-65.2973, 43.6742) -> (-63.0746, 31.0676)
  line L90 (-63.0746, 31.0676) -> (-47.7115, 33.7767)
  line L91 (-47.7115, 33.7767) -> (-49.9345, 46.3828)
  line L92 (-46.6262, 27.6222) -> (-61.9898, 24.9132)
  line L93 (-61.9898, 24.9132) -> (-59.7659, 12.3084)
  line L94 (-59.7659, 12.3084) -> (-44.4037, 15.0172)
  line L95 (-44.4037, 15.0172) -> (-46.6262, 27.6222)
  line L96 (-59.7847, 102.5157) -> (-75.1478, 99.8064)
  line L97 (-75.1478, 99.8064) -> (-72.925, 87.1998)
  line L98 (-72.925, 87.1998) -> (-57.5609, 89.9089)
  line L99 (-57.5609, 89.9089) -> (-59.7847, 102.5157)
  line L100 (-76.1309, 85.4056) -> (-91.494, 82.6968)
  line L101 (-91.494, 82.6968) -> (-89.2712, 70.0908)
  line L102 (-89.2712, 70.0908) -> (-73.9082, 72.8001)
  line L103 (-73.9082, 72.8001) -> (-76.1309, 85.4056)
  line L104 (-72.8231, 66.6451) -> (-88.1859, 63.9366)
  line L105 (-88.1859, 63.9366) -> (-85.9634, 51.3313)
  line L106 (-85.9634, 51.3313) -> (-70.5996, 54.0404)
  line L107 (-70.5996, 54.0404) -> (-72.8231, 66.6451)
  line L108 (-69.515, 47.8859) -> (-84.8781, 45.176)
  line L109 (-84.8781, 45.176) -> (-82.6553, 32.5705)
  line L110 (-82.6553, 32.5705) -> (-67.2917, 35.2795)
  line L111 (-67.2917, 35.2795) -> (-69.515, 47.8859)
  line L112 (-66.207, 29.2425) -> (-81.57, 26.534)
  line L113 (-81.57, 26.534) -> (-79.3467, 13.9282)
  line L114 (-79.3467, 13.9282) -> (-63.9834, 16.6373)
  line L115 (-63.9834, 16.6373) -> (-66.207, 29.2425)
  line L116 (-79.3644, 104.2067) -> (-94.7277, 101.4965)
  line L117 (-94.7277, 101.4965) -> (-92.5049, 88.8902)
  line L118 (-92.5049, 88.8902) -> (-77.1417, 91.6001)
  line L119 (-77.1417, 91.6001) -> (-79.3644, 104.2067)
  line L120 (-95.3622, 85.0604) -> (-110.7252, 82.351)
  line L121 (-110.7252, 82.351) -> (-108.5025, 69.7452)
  line L122 (-108.5025, 69.7452) -> (-93.1394, 72.4546)
  line L123 (-93.1394, 72.4546) -> (-95.3622, 85.0604)
  line L124 (-92.0541, 66.299) -> (-107.4174, 63.5908)
  line L125 (-107.4174, 63.5908) -> (-105.1944, 50.9855)
  line L126 (-105.1944, 50.9855) -> (-89.8313, 53.6945)
  line L127 (-89.8313, 53.6945) -> (-92.0541, 66.299)
  line L128 (-88.746, 47.5401) -> (-104.1093, 44.8302)
  line L129 (-104.1093, 44.8302) -> (-101.8865, 32.2247)
  line L130 (-101.8865, 32.2247) -> (-86.5235, 34.9335)
  line L131 (-86.5235, 34.9335) -> (-88.746, 47.5401)
  line L132 (-85.4385, 28.897) -> (-100.8012, 26.1885)
  line L133 (-100.8012, 26.1885) -> (-98.5787, 13.5834)
  line L134 (-98.5787, 13.5834) -> (-83.2154, 16.292)
  line L135 (-83.2154, 16.292) -> (-85.4385, 28.897)
  line L136 (-98.5965, 103.8614) -> (-113.9587, 101.151)
  line L137 (-113.9587, 101.151) -> (-111.7367, 88.5449)
  line L138 (-111.7367, 88.5449) -> (-96.3737, 91.2543)
  line L139 (-96.3737, 91.2543) -> (-98.5965, 103.8614)
  line L140 (-114.0738, 81.6819) -> (-129.4368, 78.972)
  line L141 (-129.4368, 78.972) -> (-127.214, 66.366)
  line L142 (-127.214, 66.366) -> (-111.8513, 69.0753)
  line L143 (-111.8513, 69.0753) -> (-114.0738, 81.6819)
  line L144 (-110.766, 62.9211) -> (-126.129, 60.2123)
  line L145 (-126.129, 60.2123) -> (-123.9062, 47.607)
  line L146 (-123.9062, 47.607) -> (-108.5432, 50.3163)
  line L147 (-108.5432, 50.3163) -> (-110.766, 62.9211)
  line L148 (-107.4579, 44.3008) -> (-122.8212, 41.5914)
  line L149 (-122.8212, 41.5914) -> (-120.5981, 28.9856)
  line L150 (-120.5981, 28.9856) -> (-105.2351, 31.695)
  line L151 (-105.2351, 31.695) -> (-107.4579, 44.3008)
  line L152 (-104.2464, 25.5889) -> (-119.6094, 22.8801)
  line L153 (-119.6094, 22.8801) -> (-117.3861, 10.2751)
  line L154 (-117.3861, 10.2751) -> (-102.0236, 12.9842)
  line L155 (-102.0236, 12.9842) -> (-104.2464, 25.5889)
  line L156 (-117.3075, 100.4816) -> (-132.6706, 97.7728)
  line L157 (-132.6706, 97.7728) -> (-130.4478, 85.1659)
  line L158 (-130.4478, 85.1659) -> (-115.0845, 87.8753)
  line L159 (-115.0845, 87.8753) -> (-117.3075, 100.4816)
  line L160 (-3.9632, 113.914) -> (-19.3262, 111.2041)
  line L161 (-19.3262, 111.2041) -> (-17.1035, 98.5986)
  line L162 (-17.1035, 98.5986) -> (-1.7404, 101.3066)
  line L163 (-1.7404, 101.3066) -> (-3.9632, 113.914)
  line L164 (-21.7231, 133.2204) -> (-140.4763, 109.2348)
  line L165 (8.6955, 133.3884) -> (8.6955, -3.1586)
  line L166 (8.6955, -3.1586) -> (8.6955, 133.3884)
  line L167 (8.6955, 133.3884) -> (-20.229, 133.3873)
  line L168 (-20.229, 133.3873) -> (-20.9817, 133.3511)
  line L169 (-20.9817, 133.3511) -> (-20.9817, 133.3521)
  line L170 (-20.9817, 133.3521) -> (-21.7239, 133.2209)
  line L171 (-21.7239, 133.2209) -> (-140.4763, 109.2346)
  line L172 (-140.4763, 109.2346) -> (-141.1965, 109.0115)
  line L173 (-141.1965, 109.0115) -> (-141.8828, 108.7009)
  line L174 (-141.8828, 108.7009) -> (-141.8828, 108.7014)
  line L175 (-141.8828, 108.7014) -> (-142.5242, 108.3067)
  line L176 (-142.5242, 108.3067) -> (-142.5242, 108.3061)
  line L177 (-142.5242, 108.3061) -> (-143.1118, 107.8333)
  line L178 (-143.1118, 107.8333) -> (-143.1118, 107.8344)
  line L179 (-143.1118, 107.8344) -> (-143.6336, 107.2928)
  line L180 (-143.6336, 107.2928) -> (-143.6349, 107.2917)
  line L181 (-143.6349, 107.2917) -> (-144.0863, 106.6879)
  line L182 (-144.0863, 106.6879) -> (-144.4591, 106.0334)
  line L183 (-144.4591, 106.0334) -> (-144.7456, 105.3362)
  line L184 (-144.7456, 105.3362) -> (-144.9427, 104.6096)
  line L185 (-144.9427, 104.6096) -> (-144.9427, 104.6107)
  line L186 (-144.9427, 104.6107) -> (-145.048, 103.8646)
  line L187 (-145.048, 103.8646) -> (-145.0472, 103.864)
  line L188 (-145.0472, 103.864) -> (-145.0583, 103.11)
  line L189 (-145.0583, 103.11) -> (-145.0589, 103.111)
  line L190 (-145.0589, 103.111) -> (-144.975, 102.3628)
  line L191 (-144.975, 102.3628) -> (-127.2429, 1.7986)
  line L192 (-127.2429, 1.7986) -> (-127.0661, 1.0668)
  line L193 (-127.0661, 1.0668) -> (-126.7981, 0.3622)
  line L194 (-126.7981, 0.3622) -> (-126.4438, -0.3029)
  line L195 (-126.4438, -0.3029) -> (-126.0097, -0.9189)
  line L196 (-126.0097, -0.9189) -> (-125.5025, -1.4745)
  line L197 (-125.5025, -1.4745) -> (-125.5019, -1.4745)
  line L198 (-125.5019, -1.4745) -> (-124.9275, -1.9627)
  line L199 (-124.9275, -1.9627) -> (-124.2975, -2.3757)
  line L200 (-124.2975, -2.3757) -> (-123.6194, -2.7064)
  line L201 (-123.6194, -2.7064) -> (-122.9064, -2.9488)
  line L202 (-122.9064, -2.9488) -> (-122.9072, -2.9488)
  line L203 (-122.9072, -2.9488) -> (-122.1692, -3.1009)
  line L204 (-122.1692, -3.1009) -> (-121.4181, -3.1586)
  line L205 (8.6955, -3.1586) -> (-121.4181, -3.1586)
  line L206 (-121.4181, -3.1586) -> (8.6955, -3.1586)
  line L207 (-134.2377, 110.4821) -> (-133.7178, 110.5874)
  line L208 (-133.7178, 110.5874) -> (-131.59, 111.0168)
  line L209 (-131.59, 111.0168) -> (-125.5257, 112.2415)
  line L210 (-125.5257, 112.2415) -> (-118.4886, 113.6621)
  line L211 (-118.4886, 113.6621) -> (-117.334, 113.8957)
  line L212 (-117.334, 113.8957) -> (-115.4967, 114.2667)
  line L213 (-115.4967, 114.2667) -> (-100.9499, 117.2041)
  line L214 (-100.9499, 117.2041) -> (-68.1818, 123.8213)
  line L215 (-68.1818, 123.8213) -> (-52.8323, 126.9209)
  line L216 (-52.8323, 126.9209) -> (-51.7977, 127.1302)
  line L217 (-51.7977, 127.1302) -> (-43.0514, 128.8965)
  line L218 (-43.0514, 128.8965) -> (-42.8987, 128.9269)
  line L219 (-42.8987, 128.9269) -> (-35.4137, 130.4385)
  line L220 (-35.4137, 130.4385) -> (-34.3622, 130.651)
  line L221 (-34.3622, 130.651) -> (-30.6435, 131.4019)
  line L222 (-30.6435, 131.4019) -> (-30.4964, 131.4318)
  line L223 (-30.4964, 131.4318) -> (-27.8445, 131.967)
  line L224 (-27.8445, 131.967) -> (-27.7005, 131.9959)
  line L225 (-27.7005, 131.9959) -> (-25.0462, 132.5322)
  line L226 (-25.0462, 132.5322) -> (-24.8991, 132.5615)
  line L227 (-24.8991, 132.5615) -> (-22.2581, 133.0949)
  line L228 (-22.2581, 133.0949) -> (-22.1107, 133.1243)
  line L229 (-22.1107, 133.1243) -> (-21.7247, 133.2024)
  line L230 (-21.7247, 133.2024) -> (-21.7241, 133.2029)
  line L231 (-21.7241, 133.2029) -> (-20.9836, 133.3336)
  line L232 (-20.9836, 133.3336) -> (-20.2295, 133.3683)
  line L233 (-20.2295, 133.3683) -> (-19.0293, 133.3683)
  line L234 (-19.0293, 133.3683) -> (-18.1284, 133.3683)
  line L235 (-18.1284, 133.3683) -> (-6.2166, 133.3693)
  line L236 (-6.2166, 133.3693) -> (-5.2006, 133.3693)
  line L237 (-5.2006, 133.3693) -> (-2.6458, 133.3693)
  line L238 (-2.6458, 133.3693) -> (6.4577, 133.3704)
  line L239 (6.4577, 133.3704) -> (6.6101, 133.3704)
  line L240 (6.6101, 133.3704) -> (6.7506, 133.3704)
  line L241 (6.7506, 133.3704) -> (8.6932, 133.3704)
  line L242 (8.6932, 133.3704) -> (8.6932, 130.6507)
  line L243 (8.6932, 130.6507) -> (8.6932, 100.4729)
  line L244 (8.6932, 100.4729) -> (8.6932, 99.4579)
  line L245 (8.6932, 99.4579) -> (8.6932, 65.1148)
  line L246 (8.6932, 65.1148) -> (8.6932, 32.3466)
  line L247 (8.6932, 32.3466) -> (8.6932, -0.4212)
  line L248 (8.6932, -0.4212) -> (8.6932, -3.1411)
  line L249 (8.6932, -3.1411) -> (-2.6458, -3.1411)
  line L250 (-2.6458, -3.1411) -> (-19.6038, -3.1411)
  line L251 (-19.6038, -3.1411) -> (-35.414, -3.1411)
  line L252 (-35.414, -3.1411) -> (-58.2676, -3.1411)
  line L253 (-58.2676, -3.1411) -> (-59.2836, -3.1411)
  line L254 (-59.2836, -3.1411) -> (-68.1821, -3.1411)
  line L255 (-68.1821, -3.1411) -> (-77.5727, -3.1411)
  line L256 (-77.5727, -3.1411) -> (-78.5865, -3.1411)
  line L257 (-78.5865, -3.1411) -> (-100.9499, -3.1411)
  line L258 (-100.9499, -3.1411) -> (-116.1915, -3.1411)
  line L259 (-116.1915, -3.1411) -> (-117.207, -3.1411)
  line L260 (-117.207, -3.1411) -> (-117.334, -3.1411)
  line L261 (-117.334, -3.1411) -> (-121.4168, -3.1411)
  line L262 (-121.4168, -3.1411) -> (-122.1679, -3.0829)
  line L263 (-122.1679, -3.0829) -> (-122.9032, -2.9316)
  line L264 (-122.9032, -2.9316) -> (-122.9058, -2.9311)
  line L265 (-122.9058, -2.9311) -> (-122.9048, -2.9311)
  line L266 (-122.9048, -2.9311) -> (-123.6178, -2.6892)
  line L267 (-123.6178, -2.6892) -> (-124.296, -2.358)
  line L268 (-124.296, -2.358) -> (-124.9222, -1.9476)
  line L269 (-124.9222, -1.9476) -> (-124.9259, -1.945)
  line L270 (-124.9259, -1.945) -> (-125.4138, -1.5301)
  line L271 (-125.4138, -1.5301) -> (-125.5001, -1.4573)
  line L272 (-125.5001, -1.4573) -> (-125.9321, -0.9856)
  line L273 (-125.9321, -0.9856) -> (-126.0078, -0.9025)
  line L274 (-126.0078, -0.9025) -> (-126.3465, -0.4215)
  line L275 (-126.3465, -0.4215) -> (-126.4417, -0.2855)
  line L276 (-126.4417, -0.2855) -> (-126.796, 0.3786)
  line L277 (-126.796, 0.3786) -> (-127.064, 1.0827)
  line L278 (-127.064, 1.0827) -> (-127.2418, 1.8148)
  line L279 (-127.2418, 1.8148) -> (-128.2922, 7.7708)
  line L280 (-128.2922, 7.7708) -> (-129.7371, 15.9628)
  line L281 (-129.7371, 15.9628) -> (-130.6166, 20.9505)
  line L282 (-130.6166, 20.9505) -> (-131.182, 24.1549)
  line L283 (-131.182, 24.1549) -> (-132.6266, 32.3469)
  line L284 (-132.6266, 32.3469) -> (-133.718, 38.5352)
  line L285 (-133.718, 38.5352) -> (-138.4059, 65.115)
  line L286 (-138.4059, 65.115) -> (-144.1849, 97.8831)
  line L287 (-144.1849, 97.8831) -> (-144.9731, 102.3533)
  line L288 (-144.9731, 102.3533) -> (-145.0559, 103.0933)
  line L289 (-145.0559, 103.0933) -> (-145.057, 103.101)
  line L290 (-145.057, 103.101) -> (-145.0559, 103.0999)
  line L291 (-145.0559, 103.0999) -> (-145.0451, 103.8545)
  line L292 (-145.0451, 103.8545) -> (-145.0462, 103.8556)
  line L293 (-145.0462, 103.8556) -> (-144.9419, 104.5951)
  line L294 (-144.9419, 104.5951) -> (-144.9408, 104.6012)
  line L295 (-144.9408, 104.6012) -> (-144.9408, 104.598)
  line L296 (-144.9408, 104.598) -> (-144.7427, 105.3261)
  line L297 (-144.7427, 105.3261) -> (-144.4569, 106.0223)
  line L298 (-144.4569, 106.0223) -> (-144.427, 106.0754)
  line L299 (-144.427, 106.0754) -> (-144.0839, 106.6779)
  line L300 (-144.0839, 106.6779) -> (-143.6367, 107.2764)
  line L301 (-143.6367, 107.2764) -> (-143.6327, 107.2811)
  line L302 (-143.6327, 107.2811) -> (-143.6312, 107.2822)
  line L303 (-143.6312, 107.2822) -> (-143.1136, 107.819)
  line L304 (-143.1136, 107.819) -> (-143.1097, 107.8233)
  line L305 (-143.1097, 107.8233) -> (-142.6099, 108.2244)
  line L306 (-142.6099, 108.2244) -> (-142.522, 108.2958)
  line L307 (-142.522, 108.2958) -> (-141.9767, 108.6321)
  line L308 (-141.9767, 108.6321) -> (-141.9095, 108.6734)
  line L309 (-141.9095, 108.6734) -> (-141.8807, 108.6914)
  line L310 (-141.8807, 108.6914) -> (-141.7778, 108.7379)
  line L311 (-141.7778, 108.7379) -> (-141.1949, 109.0014)
  line L312 (-141.1949, 109.0014) -> (-140.4747, 109.2232)
  line L313 (-140.4747, 109.2232) -> (-139.9754, 109.324)
  line L314 (-139.9754, 109.324) -> (-139.8283, 109.3539)
  line L315 (-139.8283, 109.3539) -> (-137.8132, 109.7605)
  line L316 (-137.8132, 109.7605) -> (-137.1785, 109.8886)
  line L317 (-137.1785, 109.8886) -> (-137.0311, 109.9185)
  line L318 (-137.0311, 109.9185) -> (-135.7799, 110.1712)
  line L319 (-135.7799, 110.1712) -> (-135.1211, 110.304)
  line L320 (-135.1211, 110.304) -> (-134.384, 110.453)
  line L321 (-134.384, 110.453) -> (-134.3321, 110.4638)
  line L322 (-134.3321, 110.4638) -> (-134.2377, 110.4821)
  line L323 (-84.0589, 40.5387) -> (-82.655, 32.5787)
  line L324 (-82.655, 32.5787) -> (-68.1818, 35.1298)
  line L325 (-68.1818, 35.1298) -> (-67.2917, 35.2867)
  line L326 (-67.2917, 35.2867) -> (-68.1818, 40.3326)
  line L327 (-68.1818, 40.3326) -> (-68.2183, 40.5387)
  line L328 (-68.2183, 40.5387) -> (-69.515, 47.8896)
  line L329 (-69.515, 47.8896) -> (-84.5661, 45.2358)
  line L330 (-84.5661, 45.2358) -> (-84.8778, 45.1808)
  line L331 (-84.8778, 45.1808) -> (-84.7818, 44.6349)
  line L332 (-84.7818, 44.6349) -> (-84.5664, 43.4123)
  line L333 (-84.5664, 43.4123) -> (-84.0589, 40.5387)
  line L334 (-100.9497, 90.4409) -> (-96.3729, 91.2482)
  line L335 (-96.3729, 91.2482) -> (-97.5431, 97.8829)
  line L336 (-97.5431, 97.8829) -> (-98.5957, 103.8511)
  line L337 (-98.5957, 103.8511) -> (-100.9497, 103.4357)
  line L338 (-100.9497, 103.4357) -> (-109.1417, 101.9913)
  line L339 (-109.1417, 101.9913) -> (-109.2115, 101.9789)
  line L340 (-109.2115, 101.9789) -> (-113.9576, 101.1423)
  line L341 (-113.9576, 101.1423) -> (-113.9441, 101.0658)
  line L342 (-113.9441, 101.0658) -> (-113.383, 97.8831)
  line L343 (-113.383, 97.8831) -> (-111.9389, 89.6908)
  line L344 (-111.9389, 89.6908) -> (-111.7354, 88.5388)
  line L345 (-111.7354, 88.5388) -> (-109.1414, 88.9963)
  line L346 (-109.1414, 88.9963) -> (-105.2023, 89.6908)
  line L347 (-105.2023, 89.6908) -> (-100.9497, 90.4409)
  line L348 (-71.9137, 81.0916) -> (-70.5411, 73.307)
  line L349 (-70.5411, 73.307) -> (-69.8188, 69.2108)
  line L350 (-69.8188, 69.2108) -> (-69.691, 68.4869)
  line L351 (-69.691, 68.4869) -> (-68.1821, 68.753)
  line L352 (-68.1821, 68.753) -> (-54.3272, 71.1957)
  line L353 (-54.3272, 71.1957) -> (-54.6994, 73.3071)
  line L354 (-54.6994, 73.3071) -> (-56.1451, 81.4988)
  line L355 (-56.1451, 81.4988) -> (-56.551, 83.7994)
  line L356 (-56.551, 83.7994) -> (-68.1821, 81.7494)
  line L357 (-68.1821, 81.7494) -> (-69.6053, 81.4988)
  line L358 (-69.6053, 81.4988) -> (-71.9137, 81.0916)
  line L359 (-92.7579, 46.8363) -> (-100.9499, 45.3919)
  line L360 (-100.9499, 45.3919) -> (-104.109, 44.835)
  line L361 (-104.109, 44.835) -> (-104.0733, 44.6349)
  line L362 (-104.0733, 44.6349) -> (-103.351, 40.5389)
  line L363 (-103.351, 40.5389) -> (-101.9059, 32.3469)
  line L364 (-101.9059, 32.3469) -> (-101.886, 32.2329)
  line L365 (-101.886, 32.2329) -> (-101.2394, 32.3469)
  line L366 (-101.2394, 32.3469) -> (-100.9499, 32.398)
  line L367 (-100.9499, 32.398) -> (-86.523, 34.9409)
  line L368 (-86.523, 34.9409) -> (-87.5101, 40.5387)
  line L369 (-87.5101, 40.5387) -> (-88.233, 44.6347)
  line L370 (-88.233, 44.6347) -> (-88.5939, 46.6826)
  line L371 (-88.5939, 46.6826) -> (-88.6619, 47.0673)
  line L372 (-88.6619, 47.0673) -> (-88.7457, 47.5435)
  line L373 (-88.7457, 47.5435) -> (-92.7579, 46.8363)
  line L374 (-36.3257, 98.5909) -> (-36.2008, 97.8829)
  line L375 (-36.2008, 97.8829) -> (-35.4433, 93.5876)
  line L376 (-35.4433, 93.5876) -> (-35.4137, 93.4191)
  line L377 (-35.4137, 93.4191) -> (-34.1027, 85.9848)
  line L378 (-34.1027, 85.9848) -> (-19.0296, 88.6426)
  line L379 (-19.0296, 88.6426) -> (-18.7404, 88.6936)
  line L380 (-18.7404, 88.6936) -> (-18.9164, 89.6906)
  line L381 (-18.9164, 89.6906) -> (-19.0296, 90.3335)
  line L382 (-19.0296, 90.3335) -> (-20.3605, 97.8829)
  line L383 (-20.3605, 97.8829) -> (-20.9624, 101.2976)
  line L384 (-20.9624, 101.2976) -> (-35.4134, 98.7515)
  line L385 (-35.4134, 98.7515) -> (-36.3257, 98.5909)
  line L386 (-56.9434, 105.6722) -> (-55.5696, 97.8831)
  line L387 (-55.5696, 97.8831) -> (-55.308, 96.398)
  line L388 (-55.308, 96.398) -> (-51.7977, 97.0177)
  line L389 (-51.7977, 97.0177) -> (-46.8892, 97.8831)
  line L390 (-46.8892, 97.8831) -> (-43.6057, 98.4623)
  line L391 (-43.6057, 98.4623) -> (-39.9447, 99.1082)